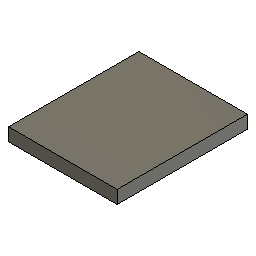
HackDeck (Autodesk Fusion 360 archive; units mm, degrees)
design "605060 LiPo Battery"
Autodesk Fusion 360 part; units mm, degrees
sketch "Sketch1" plane through (0, 0, 0) normal (0, 1, 0) x (1, 0, 0)
  line L0 (25, 30) -> (-25, 30)
  line L1 (-25, 30) -> (-25, -30)
  line L2 (-25, -30) -> (25, -30)
  line L3 (25, -30) -> (25, 30)
  line L4 (25, 30) -> (-25, -30) construction
  line L5 (-25, 30) -> (25, -30) construction
  dimension "d1" = 50
  dimension "d2" = 60
  constraint horizontal L0
  constraint perpendicular L0 L1
  constraint parallel L0 L2
  constraint parallel L1 L3
  constraint coincident L4 origin
  constraint coincident L5 origin
  measures "d1" distance of L1.end L2.end
  measures "d2" distance of L0.end L1.end
extrude "Extrude1" add sketch "Sketch1" along normal blind 6

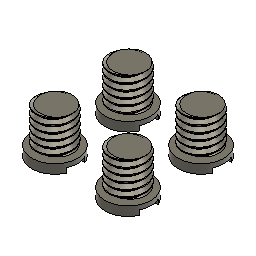
design "Screws"
Autodesk Fusion 360 part; units mm, degrees
sketch "Sketch1" plane through (0, 0, 0) normal (0, 1, 0) x (1, 0, 0)
  circle A0 centre (0, 0) radius 1.6215
  circle A1 centre (0, 0) radius 2.5
  dimension "d1" = 3.243
  dimension "d2" = 5
  constraint coincident A0.centre A1.centre
  constraint concentric A0 A1
  measures "d1" diameter of A0
  measures "d2" diameter of A1
extrude "Extrude1" add sketch "Sketch1" along normal blind 5 contours A0 makes body 1
extrude "Extrude2" add sketch "Sketch1" along normal blind 1 bodies 1
thread "Thread1" "ISO Metric profile 4.0 M4x0.7 M4x0.7 6g" major diameter 3.908 minor diameter 3.111 pitch 0.7 angle 60 modelled right hand crest width 0.1017 on face at (1.6134, 2.3333, 0.1614) crest through (1.954, 0.825, 0) on bodies 1
sketch "Sketch2" plane through (0, 0, 0) normal (0, 1, 0) x (1, 0, 0)
  line L0 (2.9915, 1) -> (-2.9915, 1)
  line L1 (-2.9915, 1) -> (-2.9915, -1)
  line L2 (-2.9915, -1) -> (2.9915, -1)
  line L3 (2.9915, -1) -> (2.9915, 1)
  line L4 (2.9915, 1) -> (-2.9915, -1) construction
  line L5 (-2.9915, 1) -> (2.9915, -1) construction
  dimension "d9" = 2
  constraint horizontal L0
  constraint perpendicular L0 L1
  constraint parallel L0 L2
  constraint parallel L1 L3
  constraint coincident L4 origin
  constraint coincident L5 origin
  measures "d9" distance of L0.end L1.end
extrude "Extrude3" cut sketch "Sketch2" along normal blind 0.5 bodies 1
copy_body "CopyPasteBodies3" bodies 1 makes body 2
move_body "Move3" bodies 2 to x (1, 0, 0) y (0, 1, 0) z (0, 0, 1) at (0, 0, -8)
copy_body "CopyPasteBodies4" bodies 2 1 makes body 3 makes body 4
move_body "Move4" bodies 3 4 to x (1, 0, 0) y (0, 1, 0) z (0, 0, 1) at (8, 0, 0)
